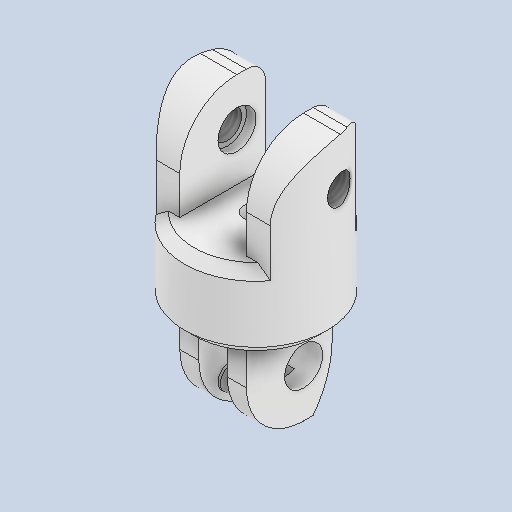
# Autodesk Inventor part: Lil_2
Saved by Autodesk Inventor 2022 (Build 260153000, 153)
## iProperties
Created: 2023-01-15
Part Number: Lil_2
Material: ABS Plastic
Document SubType Name: Modeling
Designer: 48735
Density: 1.06 g/cm^3
Appearance: Smooth - White
Author: 48735
Autodesk Inventor part; units mm, degrees
ref_plane "YZ Plane" through (0, 0, 0) normal (1, 0, 0) x (0, 1, 0)
ref_plane "XZ Plane" through (0, 0, 0) normal (0, 1, 0) x (-1, 0, 0)
ref_plane "XY Plane" through (0, 0, 0) normal (0, 0, 1) x (1, 0, 0)
sketch "Sketch1" plane through (0, 0, 0) normal (0, 1, 0) x (-1, 0, 0)
  circle A0 centre (0, 0) radius 7.5
  line L0 (3.5, 0) -> (3.5, -4.5)
  line L1 (3.5, -4.5) -> (1.5, -4.5)
  line L2 (1.5, -2.5) -> (1.5, 0)
  line L3 (3.5, 0) -> (3.5, 4.5)
  line L4 (3.5, 4.5) -> (1.5, 4.5)
  line L5 (1.5, 4.5) -> (1.5, 0)
  line L6 (-1.5, 0) -> (-1.5, 4.5)
  line L7 (-1.5, 4.5) -> (-3.5, 4.5)
  line L8 (-3.5, 4.5) -> (-3.5, 0)
  line L9 (-3.5, -4.5) -> (-3.5, 0)
  line L10 (-3.5, -4.5) -> (-1.5, -4.5)
  line L11 (-1.5, -2.5) -> (-1.5, 0)
  line L12 (3.5, -4.5) -> (3.5, -2.5)
  line L13 (1.5, -2.5) -> (-1.5, -2.5)
  line L14 (-3.5, -4.5) -> (3.5, -4.5)
  constraints: 30 end point, 7 perpendicular, 5 point on line, 3 collinear, 1 centre point, 1 coincident, 1 parallel, 1 vertical
extrude "Extrusion1" add sketch "Sketch1" along normal blind 10 contours L0 L1 L14 L10 L9 L8 L7 L6 L11 L13 L2 L5 L4 L3
fillet "Fillet1" radius 6 2 edges at (2.5, 0, 4.5) (-2.5, 0, 4.5)
fillet "Fillet2" radius 10 3 edges at (-2.5, 0, -4.5) (0, 0, -4.5) (2.5, 0, -4.5)
sketch "Sketch2" plane through (0, 10, 0) normal (0, 1, 0) x (1, 0, 0)
  circle A0 centre (0, 0) radius 7.5
  circle A1 centre (0, 0) radius 1.25
  dimension "d12" = 15
  dimension "d13" = 2.5
  constraints: 2 centre point, 2 coincident
  measures "d12" diameter of A0
  measures "d13" diameter of A1
extrude "Extrusion2" add sketch "Sketch2" along normal blind 1
chamfer "Chamfer1" distance 1 angle 45 1 edges at (-7.5, 10, 0)
fillet "Fillet3" radius 0.25 1 edges at (-1.25, 10, 0)
sketch "Sketch3" plane through (3.5, 0, -1.5) normal (1, 0, 0) x (0, 0, -1)
  line L0 (0, 0) -> (0, 5)
  point P0 (-1.5, 0)
  dimension "d20" = 5
  constraints: 2 end point, 1 vertical
  measures "d20" distance of L0.start L0.end
hole "Hole1" at (3.5, 5, -1.5) direction (-1, 0, 0) diameter 4 depth 10
sketch "Sketch4" plane through (1.5, 0, -2.5) normal (-1, 0, 0) x (0, 0, 1)
  line L0 (7, 6) -> (7, 10) projected
  circle A0 centre (3.75, 3) radius 1.25
  point P0 (2.5, 0)
  constraints: 1 centre point
extrude "Extrusion3" add sketch "Sketch4" along normal blind 1.5
chamfer "Chamfer2" distance 0.25 distance2 1.25 1 edges at (0, 3, 0) measured on face at (0, 3, 0.5)
sketch "Sketch5" plane through (-1.5, 0, -1.5) normal (1, 0, 0) x (0, 0, -1)
  circle A0 centre (-2.75, 3) radius 1.25 projected
  circle A1 centre (-2.75, 3) radius 1.25
  point P0 (-1.5, 0)
  constraints: 1 centre point, 1 coincident
extrude "Extrusion4" add sketch "Sketch5" along normal blind 1.5
chamfer "Chamfer3" distance 0.25 distance2 1.25 1 edges at (0, 3, 2.5) measured on face at (0, 3, 2.4)
sketch "Sketch6" plane through (0, 11, 0) normal (0, 1, 0) x (1, 0, 0)
  circle A0 centre (0, 0) radius 1.25
  circle A1 centre (0, 0) radius 1.25 projected
  circle A2 centre (0, 0) radius 7.5
  constraints: 2 centre point, 2 coincident
extrude "Extrusion5" add sketch "Sketch6" along normal blind 6
sketch "Sketch7" plane through (0, 17, 0) normal (0, 1, 0) x (1, 0, 0)
  circle A0 centre (0, 0) radius 1.25
  circle A1 centre (0, 0) radius 1.25 projected
  circle A2 centre (0, 0) radius 7.5
  constraints: 2 centre point, 2 coincident
extrude "Extrusion6" add sketch "Sketch7" along normal blind 1
sketch "Sketch10" plane through (0, 18, 0) normal (0, 1, 0) x (1, 0, 0)
  circle A0 centre (0, 0) radius 7.5
  line L0 (0, 0) -> (3.5, 0)
  line L1 (3.5, 0) -> (-3.5, 0)
  line L2 (-3.5, 0) -> (-3.5, -3.5)
  line L3 (-3.5, 0) -> (-3.5, 3.5)
  line L4 (3.5, 0) -> (3.5, -3.5)
  line L5 (3.5, 0) -> (3.5, 3.5)
  line L6 (3.5, -3.5) -> (3.5, -4.5)
  line L7 (3.5, -4.5) -> (6, -4.5)
  line L8 (3.5, 3.5) -> (3.5, 4.5)
  line L9 (3.5, 4.5) -> (6, 4.5)
  line L10 (-3.5, 3.5) -> (-3.5, 4.5)
  line L11 (-3.5, 4.5) -> (-6, 4.5)
  line L12 (-3.5, -3.5) -> (-3.5, -4.5)
  line L13 (-3.5, -4.5) -> (-6, -4.5)
  point P0 (-6.6332, -3.5)
  point P1 (-6.6332, 3.5)
  point P2 (6.6332, -3.5)
  point P3 (6.6332, 3.5)
  constraints: 28 end point, 8 point on line, 3 perpendicular, 1 coincident, 1 horizontal, 1 vertical, 10 other
extrude "Extrusion9" add sketch "Sketch10" along normal blind 10 contours A0 L7 L6 L4 L5 L8 L9 | L11 L10 L3 L2 L12 L13 A0
chamfer "Chamfer5" distance 1 angle 45 2 edges at (0, 18, 7.5) (0, 18, -7.5)
fillet "Fillet4" radius 6 2 edges at (-4.75, 28, 4.5) (4.75, 28, 4.5)
fillet "Fillet5" radius 2 2 edges at (4.75, 28, -4.5) (-4.75, 28, -4.5)
sketch "Sketch11" plane through (3.5, 18, -4.5) normal (-1, 0, 0) x (0, 0, 1)
  arc A0 (9, 4) -> (3, 10) centre (3, 4) ccw projected
  line L0 (3, 10) -> (3, 5)
  point P0 (4.5, -18)
  dimension "d63" = 5
  constraints: 2 end point, 1 vertical
  measures "d63" distance of L0.start L0.end
hole "Hole2" at (3.5, 23, -1.5) direction (1, 0, 0) diameter 3 depth 5 counterbore diameter 4 counterbore depth 1
sketch "Sketch12" plane through (-3.5, 18, 4.5) normal (1, 0, 0) x (0, 0, -1)
  arc A0 (6, 10) -> (0, 4) centre (6, 4) ccw projected
  line L0 (6, 10) -> (6, 5)
  point P0 (4.5, -18)
  dimension "d71" = 5
  constraints: 2 end point, 1 vertical
  measures "d71" distance of L0.start L0.end
hole "Hole3" at (-3.5, 23, -1.5) direction (-1, 0, 0) diameter 3 depth 5 counterbore diameter 4 counterbore depth 1
thread "Thread1" size "M3x0.5" class "6H" standard "ANSI Metric M Profile" length 6
thread "Thread2" size "M3x0.5" class "6H" standard "ANSI Metric M Profile" length 6
body "Solid1"
